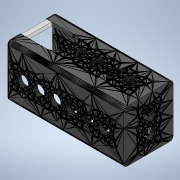
# Autodesk Inventor part: vertical_battery_holder
Saved by Autodesk Inventor 2020 (Build 240168000, 168)
## iProperties
Created: 2020-01-29
Part Number: vertical_battery_holder
Material: Generic
Document SubType Name: Modeling
Designer: jackm
Density: 1 g/cm^3
Appearance: Default
Author: jackm
Autodesk Inventor part; units mm, degrees
ref_plane "YZ Plane" through (0, 0, 0) normal (1, 0, 0) x (0, 1, 0)
ref_plane "XZ Plane" through (0, 0, 0) normal (0, 1, 0) x (-1, 0, 0)
ref_plane "XY Plane" through (0, 0, 0) normal (0, 0, 1) x (1, 0, 0)
sketch "Sketch2" plane through (-107.95, 73.766, 12.698) normal (0, -1, 0) x (1, 0, 0)
  line L0 (4.0161, 30.485) -> (-0.0057, 30.485) construction
  line L1 (-0.0057, 0) -> (4.0161, 0) construction
  line L2 (-0.0057, 30.485) -> (-0.0057, 0)
  line L3 (-0.0057, 0) -> (7.4943, 0)
  line L4 (7.4943, 0) -> (7.4943, 30.485)
  line L5 (7.4943, 30.485) -> (-0.0057, 30.485)
  point P0 (107.95, -12.698)
  dimension "d0" = 7.5
  constraints: 8 end point, 2 perpendicular, 1 point on line, 1 vertical
  measures "d0" distance of L1.start L3.end
extrude "Extrusion1" add sketch "Sketch2" against normal blind 4.25
fillet "Fillet1" radius 2 1 edges at (-107.9557, 78.016, 27.9405)
sketch "Sketch3" plane through (-63.808, 20.948, 12.862) normal (0, 1, 0) x (-1, 0, 0)
  point P0 (-63.808, -12.862)
body "Solid1"
